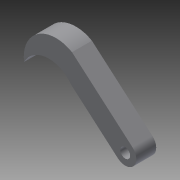
# Autodesk Inventor part: ratchet stop mk 2
Saved by Autodesk Inventor 2013 (Build 170138000, 138)
## iProperties
Created: 2014-01-06
Part Number: ratchet stop mk 2
Material: Generic
Document SubType Name: Modeling
Designer: kahohbein
Density: 1 g/cm^3
Author: kahohbein
Autodesk Inventor part; units mm, degrees
ref_plane "YZ Plane" through (0, 0, 0) normal (1, 0, 0) x (0, 1, 0)
ref_plane "XZ Plane" through (0, 0, 0) normal (0, 1, 0) x (-1, 0, 0)
ref_plane "XY Plane" through (0, 0, 0) normal (0, 0, 1) x (1, 0, 0)
sketch "Sketch1" plane through (0, 0, 0) normal (0, 0, 1) x (1, 0, 0)
  arc A0 (16.5756, -0.6685) -> (21.2023, 4.6943) centre (18.889, 2.0129) ccw
  line L0 (21.2023, 4.6943) -> (1.9212, 21.3289)
  line L1 (16.5756, -0.6685) -> (1.6942, 12.1703)
  arc A1 (1.9212, 21.3289) -> (-13.3635, 11.0028) centre (-3.1996, 12.4333) ccw
  arc A2 (1.6942, 12.1703) -> (-13.3635, 11.0028) centre (-5.482, 7.0372) ccw
  point P0 (0, 0)
  point P1 (0, 0)
  constraints: 6 point on circle, 4 end point, 3 centre point, 2 tangent, 1 parallel
extrude "Extrusion1" add sketch "Sketch1" along normal blind 6.35
sketch "Sketch2" plane through (0, 0, 6.35) normal (0, 0, 1) x (1, 0, 0)
  arc A0 (16.5756, -0.6685) -> (21.2023, 4.6943) centre (18.889, 2.0129) ccw projected
  circle A1 centre (18.889, 2.0129) radius 1.5875
  point P0 (0, 0)
  dimension "d2" = 3.175
  constraints: 1 centre point, 1 coincident
  measures "d2" diameter of A1
extrude "Extrusion2" cut sketch "Sketch2" against normal blind 6.35
body "Solid1"
